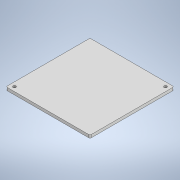
# Autodesk Inventor part: tampa caixa
Saved by Autodesk Inventor 2022 (Build 260153000, 153)
## iProperties
Created: 2022-03-13
Part Number: tampa caixa
Material: Genérico
Document SubType Name: Modeling
Designer: Hanter
Density: 1 g/cm^3
Appearance: Padrão
Author: Hanter
Autodesk Inventor part; units mm, degrees
ref_plane "YZ Plane" through (0, 0, 0) normal (1, 0, 0) x (0, 1, 0)
ref_plane "XZ Plane" through (0, 0, 0) normal (0, 1, 0) x (-1, 0, 0)
ref_plane "XY Plane" through (0, 0, 0) normal (0, 0, 1) x (1, 0, 0)
sketch "Esboço1" plane through (0, 0, 0) normal (0, 1, 0) x (-1, 0, 0)
  line L0 (-59, 59) -> (59, 59)
  line L1 (59, 59) -> (59, -59)
  line L2 (59, -59) -> (-59, -59)
  line L3 (-59, -59) -> (-59, 59)
  line L4 (-59, 59) -> (59, -59) construction
  line L5 (59, 59) -> (-59, -59) construction
  point P0 (0, 0)
  dimension "d0" = 118
  dimension "d1" = 118
  constraints: 12 end point, 2 midpoint, 2 parallel, 1 horizontal, 1 perpendicular
  measures "d0" distance of L1.end L2.end
  measures "d1" distance of L0.end L1.end
extrude "Extrusão1" add sketch "Esboço1" along normal blind 4
sketch "Esboço2" plane through (0, 0, 0) normal (0, -1, 0) x (1, 0, 0)
  line L0 (-52, -52) -> (40, -52)
  line L1 (52, -40) -> (52, 52)
  line L2 (52, 52) -> (-40, 52)
  line L3 (-52, 40) -> (-52, -52)
  line L4 (-52, -52) -> (52, 52) construction
  line L5 (52, -52) -> (-52, 52) construction
  line L6 (-40, 52) -> (-40, 44)
  line L7 (-44, 40) -> (-52, 40)
  line L8 (40, -52) -> (40, -44)
  line L9 (44, -40) -> (52, -40)
  arc A0 (-44, 40) -> (-40, 44) centre (-44, 44) ccw
  arc A1 (44, -40) -> (40, -44) centre (44, -44) ccw
  point P0 (0, 0)
  dimension "d13" = 4
  constraints: 20 end point, 4 point on circle, 4 tangent, 2 centre point, 2 midpoint, 2 parallel, 1 equal radius, 1 horizontal, 1 perpendicular
  measures "d13" radius of A0
extrude "Extrusão2" add sketch "Esboço2" along normal blind 4
fillet "Arredondamento1" radius 2 4 edges at (59, 2, 59) (59, 2, -59) (-59, 2, 59) (-59, 2, -59)
sketch "Esboço3" plane through (0, 0, 0) normal (0, -1, 0) x (1, 0, 0)
  circle A0 centre (53, -53) radius 2.005
  circle A1 centre (-53, 53) radius 2.005
  line L0 (57, -59) -> (-57, -59) projected
  line L1 (59, 57) -> (59, -57) projected
  line L2 (-59, -57) -> (-59, 57) projected
  line L3 (-57, 59) -> (57, 59) projected
  point P0 (0, 0)
  dimension "d15" = 4.01
  dimension "d16" = 4.01
  dimension "d17" = 6
  dimension "d18" = 6
  dimension "d19" = 6
  dimension "d20" = 6
  constraints: 2 centre point
  measures "d15" diameter of A0
  measures "d16" diameter of A1
  measures "d17" distance from line of L0 A0.centre
  measures "d18" distance from line of L1 A0.centre
  measures "d19" distance from line of L2 A1.centre
  measures "d20" distance from line of L3 A1.centre
extrude "Extrusão3" cut sketch "Esboço3" against normal blind 4
